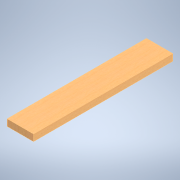
# Autodesk Inventor part: Dip Beams
Saved by Autodesk Inventor 2021 (Build 250183000, 183)
## iProperties
Created: 2020-12-20
Part Number: Dip Beams
Material: Wood (Oak)
Document SubType Name: Modeling
Designer: Jawad
Density: 0.76 g/cm^3
Appearance: Yellow Pine - Solid Stained Dark No Gloss
Author: Jawad
Autodesk Inventor part; units mm, degrees
ref_plane "YZ Plane" through (0, 0, 0) normal (1, 0, 0) x (0, 1, 0)
ref_plane "XZ Plane" through (0, 0, 0) normal (0, 1, 0) x (-1, 0, 0)
ref_plane "XY Plane" through (0, 0, 0) normal (0, 0, 1) x (1, 0, 0)
sketch "Dip beams" plane through (0, 0, 0) normal (0, 0, 1) x (1, 0, 0)
  line L0 (-98.1627, 77.231) -> (176.8373, 77.231)
  line L1 (176.8373, 77.231) -> (176.8373, 8.481)
  line L2 (176.8373, 8.481) -> (-98.1627, 8.481)
  line L3 (-98.1627, 8.481) -> (-98.1627, 77.231)
  point P0 (0, 0)
  dimension "d0" = 275
  dimension "d1" = 68.75
  constraints: 8 end point, 2 parallel, 1 horizontal, 1 perpendicular
  measures "d0" distance of L0.start L0.end
  measures "d1" distance of L0.end L1.end
extrude "Extrusion1" add sketch "Dip beams" along normal blind 1450
equation "\"d1\" = 0.25 * d0"
body "Solid1"
